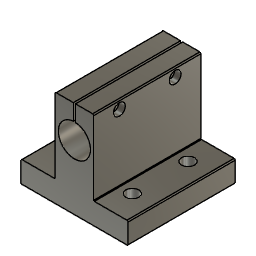
Shaft mount D15 v1 (Autodesk Fusion 360 design; units mm, degrees)
Autodesk Fusion 360 part; units mm, degrees
sketch "Sketch1" plane through (0, 0, 0) normal (0, 1, 0) x (1, 0, 0)
  line L0 (15, 0) -> (-15, 0) construction
  circle A0 centre (15, 0) radius 2.5
  circle A1 centre (-15, 0) radius 2.5
  line L1 (-25, 0) -> (25, 0)
  line L2 (25, 0) -> (25, -10)
  line L3 (-25, 0) -> (-25, -10)
  circle A2 centre (15, 0) radius 4.25
  circle A3 centre (-15, 0) radius 4.25
  line L4 (-25, -10) -> (-9, -10)
  line L5 (25, -10) -> (9, -10)
  line L6 (-9, -10) -> (-9, -45)
  line L7 (9, -10) -> (9, -45)
  line L8 (9, -45) -> (-9, -45)
  circle A4 centre (0, -30) radius 7.5
  line L9 (-0.5, -45) -> (-0.5, -37.4833)
  line L10 (0.5, -45) -> (0.5, -37.4833)
  dimension "d1" = 5
  dimension "d2" = 5
  dimension "d3" = 30
  dimension "d4" = 10
  dimension "d5" = 50
  dimension "d6" = 8.5
  dimension "d7" = 8.5
  dimension "d8" = 15
  dimension "d9" = 18
  dimension "d10" = 16
  dimension "d11" = 35
  constraint coincident L0.start A0.centre
  constraint coincident L0.end A1.centre
  constraint midpoint origin L0
  constraint parallel L0 L1
  constraint perpendicular L1 L2
  constraint perpendicular L1 L3
  constraint equal L2 L3
  constraint midpoint origin L1
  constraint concentric A0 A2
  constraint concentric A1 A3
  constraint perpendicular L3 L4
  constraint perpendicular L2 L5
  constraint perpendicular L4 L6
  constraint perpendicular L5 L7
  constraint perpendicular L6 L8
  constraint coincident L8 L9.start
  constraint coincident A4 L9.end
  constraint perpendicular L8 L9
  constraint coincident L8 L10.start
  constraint coincident A4 L10.end
  constraint perpendicular L8 L10
  measures "d1" diameter of A0
  measures "d2" diameter of A1
  measures "d3" distance of L0.start L0.end
  measures "d4" distance of L1.end L2.end
  measures "d5" distance of L1.start L1.end
  measures "d6" diameter of A2
  measures "d7" diameter of A3
  measures "d8" diameter of A4
  measures "d9" distance of L6.end L7.end
  measures "d10" distance of L2.end L5.end
  measures "d11" distance of L5.end L7.end
extrude "Extrude1" add sketch "Sketch1" along normal mid plane 50 contours A0 L1 A2 | A0 L1 | L1 L2 L3 A2 A3 L4 L5 L6 L7 L8 A4 L9 L10 | A1 L1 A3 | A1 L1 | L8 A4 L9 L10 picked at (18.6415, -0.3353) picked at (14.3891, -0.5668) picked at (-11.3492, -0.2111) picked at (-15.4919, -1.0214)
sketch "Sketch2" plane through (0, 0, 0) normal (0, 0, -1) x (1, 0, 0)
  line L0 (-25, 25) -> (-25, -25)
  line L1 (-25, -25) -> (25, -25)
  line L2 (25, -25) -> (25, 25)
  line L3 (25, 25) -> (-25, 25)
  circle A0 centre (15, -13) radius 3
  circle A1 centre (-15, -13) radius 3
  circle A2 centre (-15, 13) radius 3
  circle A3 centre (15, 13) radius 3
  dimension "d34" = 30
  dimension "d35" = 6
  constraint equal A0 A1
  constraint equal A1 A2
  constraint equal A1 A3
  measures "d34" distance of A0.centre A1.centre
  measures "d35" diameter of A1
fillet "Fillet1" radius 0.5 4 edges at (-25, 0, 10) (25, 0, 10) (9, 0, 45) (-9, 0, 45)
fillet "Fillet2" radius 0.3 2 edges at (25, 0, 0) (-25, 0, 0)
fillet "Fillet3" radius 0.3 2 edges at (-9, 0, 10) (9, 0, 10)
extrude "Extrude3" cut sketch "Sketch1" along normal mid plane 50 contours L8 A4 L9 L10
sketch "Sketch3" plane through (9, 0, 0) normal (1, 0, 0) x (0, 1, 0)
  line L0 (-25, 10.3) -> (25, 10.3)
  line L1 (25, 10.3) -> (25, 44.5)
  line L2 (25, 44.5) -> (-25, 44.5)
  line L3 (-25, 44.5) -> (-25, 10.3)
  line L4 (-24.5, 37.5) -> (24.5, 37.5) construction
  line L5 (0, 41) -> (13, 41) construction
  line L6 (0, 41) -> (-13, 41) construction
  circle A0 centre (13, 41) radius 3
  circle A1 centre (-13, 41) radius 3
  constraint perpendicular L3 L4
  constraint parallel L2 L5
  constraint parallel L5 L6
  constraint coincident L5.end A0.centre
  constraint coincident L6.end A1.centre
hole "Hole1" at (9, 13, 41) at (9, -13, 41) direction (-1, 0, 0) diameter 2.529 depth 18 tip angle 180 counterbore diameter 5.5 counterbore depth 3
thread "Thread1" "ISO Metric profile 3.0 M3x0.5 6H" major diameter 3.086 minor diameter 2.529 pitch 0.5 angle 60 resizes the face on face at (-3.3333, -14.2641, 40.9685) on face at (-3.3333, 11.7359, 40.9685) on face at (4.1667, -14.2641, 40.9685) on face at (4.1667, 11.7359, 40.9685)
sketch "Sketch4" plane through (6, 0, 0) normal (1, 0, 0) x (0, 1, 0)
  circle A0 centre (-13, 41) radius 2.75
  circle A1 centre (-13, 41) radius 1.2645
  circle A2 centre (-13, 41) radius 1.2645
  constraint concentric A0 A2
sketch "Sketch5" plane through (6, 0, 0) normal (1, 0, 0) x (0, 1, 0)
  circle A0 centre (13, 41) radius 2.75
  circle A1 centre (13, 41) radius 1.2645
  circle A2 centre (13, 41) radius 1.2645
  constraint concentric A0 A2
delete_face "DeleteFace1" 1 faces at (4.1667, -14.2641, 40.9685)
delete_face "DeleteFace2" 1 faces at (4.1667, 11.7359, 40.9685)
extrude "Extrude4" cut sketch "Sketch4" sketch "Sketch5" against normal blind 5.5 contours A1 A2 of sketch 2 contours A1 A2
extrude "Extrude5" cut sketch "Sketch2" against normal blind 10 contours A0 | A1 | A2 | A3
